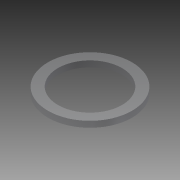
# Autodesk Inventor part: MerevitesInkrementalisFolia
Saved by Autodesk Inventor 2015 (Build 190159000, 159)
## iProperties
Created: 2014-11-14
Part Number: MerevitesInkrementalisFolia
Material: Polycarbonate, Clear
Document SubType Name: Modeling
Designer: laca
Density: 1.2 g/cm^3
Appearance: Polycarbonate - Clear
Mass: 4.75009 g
Surface Area: 34.3062 cm^2
Volume: 3.95841 cm^3
Author: laca
Autodesk Inventor part; units mm, degrees
ref_plane "YZ Plane" through (0, 0, 0) normal (1, 0, 0) x (0, 1, 0)
ref_plane "XZ Plane" through (0, 0, 0) normal (0, 1, 0) x (-1, 0, 0)
ref_plane "XY Plane" through (0, 0, 0) normal (0, 0, 1) x (1, 0, 0)
sketch "Sketch1" plane through (0, 0, 0) normal (0, 1, 0) x (-1, 0, 0)
  circle A0 centre (0, 0) radius 16
  circle A1 centre (0, 0) radius 21
  dimension "d0" = 32
  dimension "d1" = 5
  constraints: 2 centre point, 2 coincident
  measures "d0" diameter of A0
  measures "d1" radial gap between concentric circles of A1 A0
extrude "Extrusion1" add sketch "Sketch1" along normal blind 3
body "Solid1"
